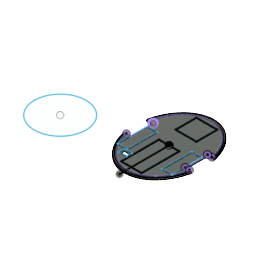
Base_Sumo (Autodesk Fusion 360 design; units mm, degrees)
Autodesk Fusion 360 part; units mm, degrees
sketch "Sketch1" plane through (0, 0, 0) normal (0, 0, 1) x (1, 0, 0)
  line L0 (-54.7772, 22.5) -> (-54.7772, -22.5)
  line L1 (-54.7772, -22.5) -> (-67.7772, -22.5)
  ellipse E0 centre (0, 0) end of major axis (-70, 0) minor radius 90
  line L2 (70, 0) -> (-70, 0) construction
  line L3 (-54.7772, 22.5) -> (-67.7772, 22.5)
  line L4 (0, 0) -> (70, 0) construction
  line L5 (0, 0) -> (0, 90) construction
  line L6 (54.7772, 22.5) -> (54.7772, -22.5)
  line L7 (54.7772, -22.5) -> (67.7772, -22.5)
  line L8 (54.7772, 22.5) -> (67.7772, 22.5)
  dimension "d2" = 45
  dimension "d29" = 13
  dimension "d30" = 70
  dimension "d31" = 90
  dimension "d32" = 13
  constraint perpendicular L0 L1
  constraint coincident E0 L2.start
  constraint coincident E0 L2.end
  constraint coincident L1.end E0
  constraint horizontal L1
  constraint perpendicular L0 L3
  constraint coincident E0 L3.end
  constraint horizontal E0.centre L4.start
  constraint coincident E0.centre L4.start
  constraint horizontal L4
  constraint perpendicular L4 L5
  constraint coincident L2.start L4.end
  constraint coincident E0 L5.end
  constraint symmetric L0.start L5 L6.start
  constraint symmetric L0.end L5 L6.end
  constraint symmetric L1.end L5 L7.end
  constraint symmetric L3.end L5 L8.end
  measures "d2" distance of L0.start L0.end
  measures "d29" distance of L0.start L3.end
  measures "d30" distance of E0.centre L2.start
  measures "d31" distance of E0.centre L5.end
  measures "d32" distance of L0.end L1.end
extrude "Extrude1" add sketch "Sketch1" along normal blind 3 contours L0 L1 E0 L3 L6 L7 L8
sketch "Sketch2" plane through (0, 0, 3) normal (0, 0, 1) x (-1, 0, 0)
  line L0 (54.7772, -22.5) -> (54.7772, 22.5)
  line L1 (67.7772, -22.5) -> (54.7772, -22.5)
  ellipse E0 centre (0, 0) end of major axis (0, 90) minor radius 70 (-67.7772, -22.5) -> (67.7772, -22.5) ccw
  line L2 (54.7772, 22.5) -> (67.7772, 22.5)
  line L3 (-54.7772, 22.5) -> (-54.7772, -22.5)
  line L4 (-54.7772, -22.5) -> (-67.7772, -22.5)
  ellipse E1 centre (0, 0) end of major axis (0, 90) minor radius 70 (67.7772, 22.5) -> (-67.7772, 22.5) ccw
  line L5 (-67.7772, 22.5) -> (-54.7772, 22.5)
  ellipse E2 centre (0, 0) end of major axis (68.5, 0) minor radius 86.5
  line L6 (-68.5, 0) -> (68.5, 0) construction
  line L7 (0, -86.5) -> (0, 86.5) construction
  ellipse E3 centre (0, 0) end of major axis (66, 0) minor radius 85
  line L8 (-66, 0) -> (66, 0) construction
  line L9 (0, -85) -> (0, 85) construction
  dimension "d33" = 137
  dimension "d34" = 173
  dimension "d35" = 132
  dimension "d36" = 170
  constraint coincident E2 L6.start
  constraint coincident E2 L6.end
  constraint coincident E2 L7.start
  constraint coincident E2 L7.end
  constraint concentric E0 E2
  constraint perpendicular L0 L6
  constraint coincident E3 L8.start
  constraint coincident E3 L8.end
  constraint coincident E3 L9.start
  constraint coincident E3 L9.end
  constraint concentric E0 E3
  constraint perpendicular L0 L8
  measures "d33" distance of E2
  measures "d35" distance of E3
extrude "Extrude2" cut sketch "Sketch2" against normal blind 1.5 contours L1 L2 E2 E3 | L1 L4 E2 E3 | L2 L5 E2 E3 | L4 L5 E2 E3
sketch "Sketch3" plane through (0, 0, 3) normal (0, 0, 1) x (-1, 0, 0)
  line L0 (21, -76) -> (-21, -76)
  line L1 (-21, -76) -> (-21, -34)
  line L2 (-21, -34) -> (21, -34)
  line L3 (21, -34) -> (21, -76)
  line L4 (63.6457, -22.5) -> (54.7772, -22.5)
  line L5 (54.7772, 22.5) -> (63.6457, 22.5)
  line L6 (54.7772, -22.5) -> (54.7772, 22.5)
  line L7 (-54.7772, 22.5) -> (-54.7772, -22.5)
  line L8 (-54.7772, -22.5) -> (-63.6457, -22.5)
  line L9 (-63.6457, 22.5) -> (-54.7772, 22.5)
  ellipse E0 centre (0, 0) end of major axis (0, 85) minor radius 66 (63.6457, 22.5) -> (-63.6457, 22.5) ccw
  ellipse E1 centre (0, 0) end of major axis (0, 85) minor radius 66 (-63.6457, -22.5) -> (63.6457, -22.5) ccw
  line L10 (-34.7974, -11.3414) -> (-54.7974, -11.3414)
  line L11 (-54.7974, -11.3414) -> (-54.7974, 48.6586)
  line L12 (-54.7974, 48.6586) -> (-34.7974, 48.6586)
  line L13 (-34.7974, 48.6586) -> (-34.7974, -11.3414)
  line L14 (54.9535, -10.6734) -> (34.9535, -10.6734)
  line L15 (34.9535, -10.6734) -> (34.9535, 49.3266)
  line L16 (34.9535, 49.3266) -> (54.9535, 49.3266)
  line L17 (54.9535, 49.3266) -> (54.9535, -10.6734)
  line L18 (-20.5, 0) -> (20.5, 0)
  line L19 (20.5, 0) -> (20.5, 76)
  line L20 (20.5, 76) -> (-20.5, 76)
  line L21 (-20.5, 76) -> (-20.5, 0)
  line L22 (38.1039, 52.22) -> (23.1039, 52.22)
  line L23 (23.1039, 52.22) -> (23.1039, 62.22)
  line L24 (23.1039, 62.22) -> (38.1039, 62.22)
  line L25 (38.1039, 62.22) -> (38.1039, 52.22)
  circle A0 centre (162.6967, 56.966) radius 52
  line L26 (0, 0) -> (0, 100)
  dimension "d21" = 42
  dimension "d22" = 42
  dimension "d37" = 20
  dimension "d38" = 60
  dimension "d39" = 20
  dimension "d40" = 60
  dimension "d41" = 41
  dimension "d42" = 76
  dimension "d43" = 15
  dimension "d44" = 10
  dimension "d45" = 104
  dimension "d46" = 100
  dimension "d47" = 20.5
  dimension "d48" = 21
  dimension "d49" = 34
  constraint horizontal L0
  constraint vertical L1
  constraint horizontal L2
  constraint vertical L3
  constraint horizontal L10
  constraint vertical L11
  constraint horizontal L12
  constraint vertical L13
  constraint horizontal L14
  constraint vertical L15
  constraint horizontal L16
  constraint vertical L17
  constraint horizontal L18
  constraint vertical L19
  constraint horizontal L20
  constraint vertical L21
  constraint horizontal L22
  constraint vertical L23
  constraint horizontal L24
  constraint vertical L25
  constraint coincident E0.centre E1.centre
  constraint perpendicular L20 L26
  constraint coincident L18 E0.centre
  measures "d21" distance of L0.start L0.end
  measures "d22" distance of L0.start L2.end
  measures "d37" distance of L10.start L10.end
  measures "d38" distance of L10.start L12.end
  measures "d39" distance of L14.end L14.start
  measures "d40" distance of L14.start L16.end
  measures "d41" distance of L18.start L18.end
  measures "d42" distance of L18.start L20.end
  measures "d43" distance of L22.start L22.end
  measures "d44" distance of L22.start L24.end
  measures "d45" diameter of A0
  measures "d46" distance of E0.centre L26.end
  measures "d47" distance of L21 L26
  measures "d48" distance of L3 L26
  measures "d49" distance of L2 E0.centre
extrude "Extrude3" cut sketch "Sketch3" against normal blind 0.5 contours L0 L1 L2 L3 | L5 L6 E0 L14 L15 L16 L17 | L7 L9 E0 L10 L11 L12 L13 | L18 L20 L21 L26 | L18 L19 L20 L26
extrude "Extrude4" cut sketch "Sketch3" against normal blind 3 contours L22 L23 L24 L25
